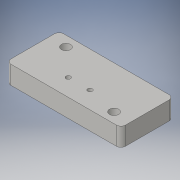
# Autodesk Inventor part: A8-0016
Saved by Autodesk Inventor 2016 SP2 (Build 200236200, 236)
## iProperties
Created: 2017-04-22
Part Number: A8-0016
Material: Generic
Document SubType Name: Modeling
Designer: EV
Density: 1 g/cm^3
Appearance: Default
Author: EV
Autodesk Inventor part; units mm, degrees
ref_plane "YZ Plane" through (0, 0, 0) normal (1, 0, 0) x (0, 1, 0)
ref_plane "XZ Plane" through (0, 0, 0) normal (0, 1, 0) x (-1, 0, 0)
ref_plane "XY Plane" through (0, 0, 0) normal (0, 0, 1) x (1, 0, 0)
sketch "Sketch1" plane through (0, 0, 0) normal (0, 1, 0) x (-1, 0, 0)
  line L0 (0, 0) -> (-50, 0)
  line L1 (-50, 0) -> (-50, -23)
  line L2 (-50, -23) -> (0, -23)
  line L3 (0, -23) -> (0, 0)
  dimension "d0" = 50
  dimension "d1" = 23
  constraints: 8 end point, 2 parallel, 1 horizontal, 1 perpendicular
  measures "d0" distance of L0.start L0.end
  measures "d1" distance of L2.end L0.start
extrude "Extrusion1" add sketch "Sketch1" along normal blind 8
sketch "Sketch2" plane through (0, 8, 0) normal (0, 1, 0) x (1, 0, 0)
  line L0 (0, 0) -> (50, 0) construction
  line L1 (50, 0) -> (50, 23) construction
  line L2 (50, 23) -> (0, 23) construction
  line L3 (0, 23) -> (0, 0) construction
  point P0 (7.5, 18.5)
  point P1 (19.5, 7.5)
  point P2 (29, 7.5)
  point P3 (42.5, 4.5)
  dimension "d5" = 4.5
  dimension "d6" = 7.5
  dimension "d7" = 7.5
  dimension "d8" = 19.5
  dimension "d9" = 9.5
  dimension "d10" = 7.5
  dimension "d11" = 4.5
  constraints: 1 horizontal alignment
  measures "d5" distance from line of L0 point (42.5, 4.5)
  measures "d6" distance from line of L0 point (19.5, 7.5)
  measures "d7" distance from line of L3 point (7.5, 18.5)
  measures "d8" distance from line of L3 point (19.5, 7.5)
  measures "d9" distance of point (19.5, 7.5) point (29, 7.5)
  measures "d10" distance from line of L1 point (42.5, 4.5)
  measures "d11" distance from line of L2 point (7.5, 18.5)
hole "Hole1" at (19.5, 8, -7.5) at (29, 8, -7.5) direction (0, -1, 0) diameter 2 end through all
hole "Hole2" at (7.5, 8, -18.5) at (42.5, 8, -4.5) direction (0, -1, 0) diameter 4 end through all
fillet "Fillet1" radius 2 4 edges at (0, 4, 0) (0, 4, -23) (50, 4, 0) (50, 4, -23)
body "Solid1"
